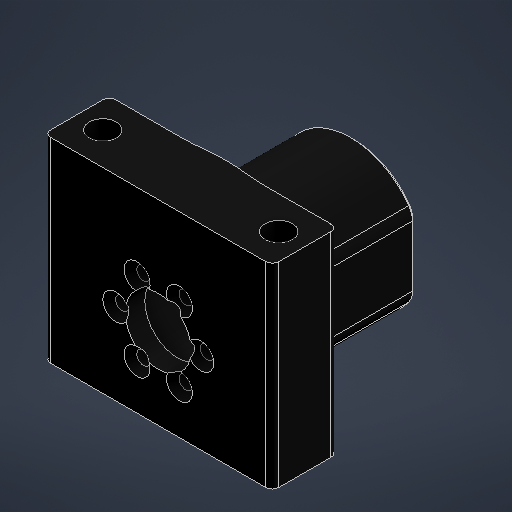
# Autodesk Inventor part: gute motorhalterung von faaaaabs
Saved by Autodesk Inventor 2025.3 (Build 293356000, 356)
## iProperties
Created: 2025-01-10
Part Number: gute motorhalterung von faaaaabs
Material: Generisch
Document SubType Name: Modeling
Designer: theod
Density: 1 g/cm^3
Appearance: Vorgabe(1)
Author: theod
Autodesk Inventor part; units mm, degrees
ref_plane "YZ Plane" through (0, 0, 0) normal (1, 0, 0) x (0, 1, 0)
ref_plane "XZ Plane" through (0, 0, 0) normal (0, 1, 0) x (-1, 0, 0)
ref_plane "XY Plane" through (0, 0, 0) normal (0, 0, 1) x (1, 0, 0)
sketch "Skizze1" plane through (0, 0, 0) normal (0, 0, 1) x (1, 0, 0)
  line L0 (-16.5, 5) -> (16.5, 5)
  line L1 (17.5, 4) -> (17.5, -4)
  line L2 (16.5, -5) -> (-16.5, -5)
  line L3 (-17.5, -4) -> (-17.5, 4)
  line L4 (-17.5, 5) -> (17.5, -5) construction
  line L5 (17.5, 5) -> (-17.5, -5) construction
  line L6 (0, 5) -> (0, -5)
  line L7 (-17.5, 0) -> (-13.5, 0)
  circle A0 centre (-13.5, 0) radius 2.1
  circle A1 centre (13.5, 0) radius 2.1
  arc A2 (-16.5, 5) -> (-17.5, 4) centre (-16.5, 4) ccw
  arc A3 (-17.5, -4) -> (-16.5, -5) centre (-16.5, -4) ccw
  arc A4 (16.5, -5) -> (17.5, -4) centre (16.5, -4) ccw
  arc A5 (17.5, 4) -> (16.5, 5) centre (16.5, 4) ccw
  point P0 (0, 0)
  dimension "d0" = 35
  dimension "d1" = 10
  dimension "d4" = 4
  dimension "d5" = 4.2
  dimension "d6" = 1
  constraints: 16 end point, 8 point on circle, 8 point on line, 8 tangent, 6 centre point, 5 midpoint, 3 equal radius, 2 horizontal, 2 parallel, 1 coincident, 1 perpendicular, 1 symmetric about line, 1 other
  measures "d0" distance of L4.end L5.end
  measures "d1" distance of L5.start L4.end
  measures "d4" distance of L7.start L7.end
  measures "d5" diameter of A0
  measures "d6" radius of A2
extrude "Extrusion1" add sketch "Skizze1" along normal mid plane 25
sketch "Skizze2" plane through (-16.5, -5, 12.5) normal (0, -1, 0) x (1, 0, 0)
  line L0 (34, -25) -> (34, 0) projected
  line L1 (0, 0) -> (-1, 0) projected
  line L2 (34, -25) -> (-1, -25)
  line L3 (-1, -25) -> (-1, 0)
  line L4 (-1, 0) -> (34, 0)
  line L5 (34, 0) -> (34, -25)
  line L6 (34, -25) -> (-1, 0) construction
  line L7 (34, 0) -> (-1, -25) construction
  circle A0 centre (16.5, -12.5) radius 8
  circle A1 centre (16.5, -12.5) radius 5
  circle A2 centre (19.75, -6.8708) radius 0.87
  circle A3 centre (23, -12.5) radius 0.87
  circle A4 centre (19.75, -18.1292) radius 0.87
  circle A5 centre (13.25, -18.1292) radius 0.87
  circle A6 centre (10, -12.5) radius 0.87
  circle A7 centre (13.25, -6.8708) radius 0.87
  point P0 (16.5, -12.5)
  point P1 (16.5, -12.5)
  constraints: 12 end point, 8 centre point, 2 parallel, 1 horizontal, 1 midpoint, 1 perpendicular
hole "Bohrung1" at (3.25, -5, 5.6292) at (6.5, -5, 0) at (3.25, -5, -5.6292) at (-3.25, -5, -5.6292) at (-6.5, -5, 0) at (-3.25, -5, 5.6292) direction (0, 1, 0) diameter 2.05 end through all countersink diameter 4 countersink angle 90
sketch "Skizze3" plane through (-16.5, 5, 12.5) normal (0, 1, 0) x (1, 0, 0)
  circle A0 centre (16.5, 12.5) radius 8.05
  circle A1 centre (16.5, 12.5) radius 5.05
  dimension "d17" = 16.1
  dimension "d18" = 10.1
  constraints: 2 centre point, 2 coincident
  measures "d17" diameter of A0
  measures "d18" diameter of A1
extrude "Extrusion2" cut sketch "Skizze3" against normal blind 7 contours A0 | A1
extrude "Extrusion3" cut sketch "Skizze3" against normal up to surface (10 mm away) contours A1
sketch "Skizze4" plane through (-16.5, 5, 12.5) normal (0, 1, 0) x (1, 0, 0)
  circle A0 centre (16.5, 12.5) radius 8.05
  circle A1 centre (16.5, 12.5) radius 11
  line L0 (27.5, 12.5) -> (26, 12.5)
  line L1 (26, 12.5) -> (26, 6.9547)
  line L2 (26, 12.5) -> (26, 18.0453)
  line L3 (5.5, 12.5) -> (7, 12.5)
  line L4 (7, 12.5) -> (7, 6.9547)
  line L5 (7, 12.5) -> (7, 18.0453)
  dimension "d23" = 22
  dimension "d30" = 1.5
  dimension "d31" = 1.5
  constraints: 12 end point, 6 point on circle, 2 centre point, 2 coincident, 2 horizontal, 2 perpendicular, 2 point on line
  measures "d23" diameter of A1
  measures "d30" distance of L0.start L0.end
  measures "d31" distance of L3.start L3.end
extrude "Extrusion4" add sketch "Skizze4" along normal blind 20 contours L2 L1 A1 L4 L5
fillet "Rundung1" radius 3 4 edges at (9.5, 15, 5.5453) (9.5, 15, -5.5453) (-9.5, 15, -5.5453) (-9.5, 15, 5.5453)
chamfer "Fasen1" distance 0.5 angle 45 9 edges at (-8.05, 25, 0) (0, 25, 11) (9.3559, 25, 5.5822) (9.5, 25, 0) (9.3559, 25, -5.5822) (0, 25, -11) (-9.3559, 25, -5.5822) (-9.5, 25, 0) (-9.3559, 25, 5.5822)
fillet "Rundung2" radius 3 8 edges at (-9.3559, 5, 5.5822) (-9.5, 5, 0) (-9.3559, 5, -5.5822) (0, 5, -11) (9.3559, 5, -5.5822) (9.5, 5, 0) (9.3559, 5, 5.5822) (0, 5, 11)
sketch "Skizze5" plane through (0, 0, 12.5) normal (0, 0, 1) x (1, 0, 0)
  arc A0 (-17.5, -4) -> (-16.5, -5) centre (-16.5, -4) ccw projected
  line L0 (-16.5, -5) -> (16.5, -5) projected
  arc A1 (16.5, -5) -> (17.5, -4) centre (16.5, -4) ccw projected
  line L1 (17.5, -4) -> (17.5, 4) projected
  arc A2 (17.5, 4) -> (16.5, 5) centre (16.5, 4) ccw projected
  line L2 (16.5, 5) -> (6.3048, 5) projected
  spline S0 degree 8 poles (6.3048, 5) (6.2653, 5) (6.2259, 5.0001) (6.1864, 5.0004) (6.1469, 5.0007) (6.1075, 5.0012) (6.068, 5.0018) (6.0286, 5.0024) (5.676, 5.0095) (5.3628, 5.0225) (5.0497, 5.041) (4.7366, 5.064) (4.4236, 5.0905) (4.1106, 5.1193) (3.7975, 5.1495) (3.0505, 5.2223) (2.6165, 5.2652) (2.1819, 5.3061) (1.7464, 5.3425) (1.3101, 5.3717) (0.8731, 5.3919) (0.4356, 5.402) (-0.4384, 5.4019) (-0.8748, 5.3918) (-1.3108, 5.3716) (-1.746, 5.3425) (-2.1804, 5.3062) (-2.614, 5.2654) (-3.047, 5.2226) (-3.5136, 5.1771) (-3.5476, 5.1738) (-3.5816, 5.1705) (-3.6156, 5.1672) (-3.6496, 5.1639) (-3.6836, 5.1606) (-3.7176, 5.1574) (-4.0709, 5.1235) (-4.3899, 5.0939) (-4.709, 5.0665) (-5.0281, 5.0423) (-5.3474, 5.0223) (-5.6666, 5.0079) (-5.9858, 5) (-6.3048, 5) knots 0 0 0 0 0 0 0 0 0 0.025118 0.025118 0.025118 0.025118 0.025118 0.025118 0.025118 0.224353 0.224353 0.224353 0.224353 0.224353 0.224353 0.224353 0.500151 0.500151 0.500151 0.500151 0.500151 0.500151 0.500151 0.775279 0.775279 0.775279 0.775279 0.775279 0.775279 0.775279 0.79691 0.79691 0.79691 0.79691 0.79691 0.79691 0.79691 1 1 1 1 1 1 1 1 1 projected
  line L3 (-6.3048, 5) -> (-16.5, 5) projected
  arc A3 (-16.5, 5) -> (-17.5, 4) centre (-16.5, 4) ccw projected
  line L4 (-17.5, 4) -> (-17.5, -4) projected
  circle A4 centre (13.5, 0) radius 2.1 projected
  circle A5 centre (-13.5, 0) radius 2.1 projected
  point P0 (0, 0)
  constraints: 1 horizontal alignment
extrude "Extrusion6" add sketch "Skizze5" along normal blind 5
